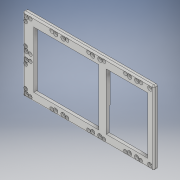
# Autodesk Inventor part: 30_CUBE_openSIM_Cagelid
Saved by Autodesk Inventor 2019 (Build 230136000, 136)
## iProperties
Created: 2020-08-12
Part Number: 30_CUBE_openSIM_Cagelid
Material: Generic
Document SubType Name: Modeling
Designer: wanghaoran
Density: 1 g/cm^3
Appearance: Default
Author: wanghaoran
Autodesk Inventor part; units mm, degrees
ref_plane "YZ Plane" through (0, 0, 0) normal (1, 0, 0) x (0, 1, 0)
ref_plane "XZ Plane" through (0, 0, 0) normal (0, 1, 0) x (-1, 0, 0)
ref_plane "XY Plane" through (0, 0, 0) normal (0, 0, 1) x (1, 0, 0)
sketch "Sketch1" plane through (0, 0, 0) normal (0, 0, 1) x (1, 0, 0)
  line L0 (0, 0) -> (177.7, 0)
  line L1 (177.7, 0) -> (177.7, 99.8)
  line L2 (177.7, 99.8) -> (0, 99.8)
  line L3 (0, 99.8) -> (0, 0)
  dimension "d0" = 177.7
  dimension "d1" = 99.8
  constraints: 8 end point, 2 parallel, 1 horizontal, 1 perpendicular
  measures "d0" distance of L2.end L1.end
  measures "d1" distance of L1.end L0.end
extrude "Extrusion1" add sketch "Sketch1" along normal blind 5.079
sketch "Sketch3" plane through (0, 0, 5.079) normal (0, 0, 1) x (1, 0, 0)
  circle A0 centre (172.7, 94.9) radius 1.45 projected
  circle A1 centre (104.9, 94.9) radius 1.45 projected
  circle A2 centre (4.9, 94.9) radius 1.45 projected
  circle A3 centre (4.9, 4.9) radius 1.6 projected
  circle A4 centre (172.7, 4.9) radius 1.45 projected
  circle A5 centre (4.9, 44.9) radius 1.6 projected
  arc A6 (144.1319, 97.8) -> (145.6681, 97.8) centre (144.9, 94.9) ccw projected
  arc A7 (154.1319, 97.8) -> (155.6681, 97.8) centre (154.9, 94.9) ccw projected
  arc A8 (94.1319, 97.8) -> (95.6681, 97.8) centre (94.9, 94.9) ccw projected
  arc A9 (54.1319, 97.8) -> (55.6681, 97.8) centre (54.9, 94.9) ccw projected
  arc A10 (44.1319, 97.8) -> (45.6681, 97.8) centre (44.9, 94.9) ccw projected
  arc A11 (2, 54.1319) -> (2, 55.6681) centre (4.9, 54.9) ccw projected
  arc A12 (2, 44.1319) -> (2, 45.6681) centre (4.9, 44.9) ccw projected
  arc A13 (45.6681, 2) -> (44.1319, 2) centre (44.9, 4.9) ccw projected
  arc A14 (55.6681, 2) -> (54.1319, 2) centre (54.9, 4.9) ccw projected
  arc A15 (95.6681, 2) -> (94.1319, 2) centre (94.9, 4.9) ccw projected
  arc A16 (105.6681, 2) -> (104.1319, 2) centre (104.9, 4.9) ccw projected
  arc A17 (145.6681, 2) -> (144.1319, 2) centre (144.9, 4.9) ccw projected
  arc A18 (155.6681, 2) -> (154.1319, 2) centre (154.9, 4.9) ccw projected
hole "Hole1" at (172.7, 4.9, 5.079) at (172.7, 94.9, 5.079) at (4.9, 94.9, 5.079) at (4.9, 44.9, 5.079) at (4.9, 4.9, 5.079) at (144.9, 94.9, 5.079) at (154.9, 94.9, 5.079) at (154.9, 4.9, 5.079) at (144.9, 4.9, 5.079) at (104.9, 4.9, 5.079) at (94.9, 4.9, 5.079) at (104.9, 94.9, 5.079) at (94.9, 94.9, 5.079) at (54.9, 94.9, 5.079) at (44.9, 94.9, 5.079) at (54.9, 4.9, 5.079) at (44.9, 4.9, 5.079) at (4.9, 54.9, 5.079) direction (0, 0, -1) diameter 2.9 depth 12 tip angle 118 counterbore diameter 6 counterbore depth 2.5
sketch "Sketch5" plane through (0, 0, 0) normal (0, 0, -1) x (-1, 0, 0)
  line L0 (-15, 11.5) -> (-169.7, 11.5)
  line L1 (-169.7, 11.5) -> (-169.7, 88.3)
  line L2 (-169.7, 88.3) -> (-15, 88.3)
  line L3 (-15, 88.3) -> (-15, 11.5)
  line L4 (0, 99.8) -> (0, 0) projected
  line L5 (-103.5, 88.3) -> (-113.5, 88.3)
  line L6 (-113.5, 88.3) -> (-113.5, 11.5)
  line L7 (-113.5, 11.5) -> (-103.5, 11.5)
  line L8 (-103.5, 11.5) -> (-103.5, 88.3)
  dimension "d28" = 154.7
  dimension "d29" = 76.8
  dimension "d49" = 15
  dimension "d58" = 10
  dimension "d59" = 76.8
  dimension "d60" = 56.2
  constraints: 16 end point, 4 parallel, 2 horizontal, 2 perpendicular, 1 point on line
  measures "d28" distance of L1.end L2.end
  measures "d29" distance of L0.end L1.end
  measures "d49" distance between parallel lines of L3 L4
  measures "d58" distance of L7.end L6.end
  measures "d59" distance of L6.end L5.end
  measures "d60" distance between parallel lines of L1 L6
extrude "Extrusion4" cut sketch "Sketch5" against normal through all contours L0 L8 L2 L3 | L0 L1 L2 L6
fillet "Fillet1" radius 2 8 edges at (88.85, 0, 5.079) (0, 49.9, 5.079) (177.7, 49.9, 5.079) (88.85, 99.8, 5.079) (177.7, 0, 2.5395) (177.7, 99.8, 2.5395) (0, 0, 2.5395) (0, 99.8, 2.5395)
sketch "Sketch7" plane through (103.5, 11.5, 0) normal (-1, 0, 0) x (0, 0, 1)
  circle A0 centre (-19.9999, 12.5) radius 13.3985 projected
  line L0 (-1.6569, 33.566) -> (-38.3429, 33.566)
  line L1 (-38.3429, 33.566) -> (-41.0659, 30.843)
  line L2 (-41.0659, 30.843) -> (-41.0659, -5.843)
  line L3 (-41.0659, -5.843) -> (-38.3429, -8.566)
  line L4 (-38.3429, -8.566) -> (-1.6569, -8.566)
  line L5 (-1.6569, -8.566) -> (1.0661, -5.843)
  line L6 (1.0661, -5.843) -> (1.0661, 30.843)
  line L7 (1.0661, 30.843) -> (-1.6569, 33.566)
  point P0 (0, -11.5)
  constraints: 16 end point
extrude "Extrusion6" cut sketch "Sketch7" against normal up to surface (154.7 mm away) from surface at 88.5
sketch "Sketch8" plane through (0, 0, 5.079) normal (0, 0, 1) x (1, 0, 0)
  circle A0 centre (160.4, 4.1) radius 2.65 projected
  circle A1 centre (189.4, 4.1) radius 2.65 projected
  circle A2 centre (154.1, 10.4) radius 2.65 projected
  circle A3 centre (195.7, 10.4) radius 2.65 projected
  circle A4 centre (145.7, 10.4) radius 2.65 projected
  circle A5 centre (139.4, 4.1) radius 2.65 projected
  circle A6 centre (110.4, 4.1) radius 2.65 projected
  circle A7 centre (89.4, 4.1) radius 2.65 projected
  circle A8 centre (60.4, 4.1) radius 2.65 projected
  circle A9 centre (39.4, 4.1) radius 2.65 projected
  circle A10 centre (10.4, 4.1) radius 2.65 projected
  circle A11 centre (4.1, 10.4) radius 2.65 projected
  circle A12 centre (4.1, 39.4) radius 2.65 projected
  circle A13 centre (10.4, 45.7) radius 2.65 projected
  circle A14 centre (4.1, 89.4) radius 2.65 projected
  circle A15 centre (10.4, 95.7) radius 2.65 projected
  circle A16 centre (39.4, 95.7) radius 2.65 projected
  circle A17 centre (60.4, 95.7) radius 2.65 projected
  circle A18 centre (89.4, 95.7) radius 2.65 projected
  circle A19 centre (110.4, 95.7) radius 2.65 projected
  circle A20 centre (139.4, 95.7) radius 2.65 projected
  circle A21 centre (160.4, 95.7) radius 2.65 projected
  circle A22 centre (189.4, 95.7) radius 2.65 projected
  circle A23 centre (4.1, 60.4) radius 2.65 projected
  circle A24 centre (10.4, 54.1) radius 2.65 projected
  circle A25 centre (4.1, 89.4) radius 2.45
  circle A26 centre (10.4, 95.7) radius 2.45
  circle A27 centre (4.1, 60.4) radius 2.45
  circle A28 centre (10.4, 54.1) radius 2.45
  circle A29 centre (10.4, 45.7) radius 2.45
  circle A30 centre (4.1, 39.4) radius 2.45
  circle A31 centre (4.1, 10.4) radius 2.45
  circle A32 centre (10.4, 4.1) radius 2.45
  circle A33 centre (39.4, 4.1) radius 2.45
  line L0 (103.5, 11.5) -> (15, 11.5) projected
  line L1 (15, 11.5) -> (25, 11.5)
  circle A34 centre (60.4, 4.1) radius 2.45
  circle A35 centre (89.4, 4.1) radius 2.45
  circle A36 centre (110.4, 4.1) radius 2.45
  circle A37 centre (139.4, 4.1) radius 2.45
  circle A38 centre (160.4, 4.1) radius 2.45
  circle A39 centre (160.4, 95.7) radius 2.45
  circle A40 centre (139.4, 95.7) radius 2.45
  circle A41 centre (110.4, 95.7) radius 2.45
  circle A42 centre (89.4, 95.7) radius 2.45
  circle A43 centre (60.4, 95.7) radius 2.45
  circle A44 centre (39.4, 95.7) radius 2.45
  point P0 (0, 0)
  dimension "d69" = 0.2
  dimension "d70" = 0.2
  dimension "d71" = 4.9
  dimension "d72" = 4.9
  dimension "d73" = 4.9
  dimension "d74" = 4.9
  dimension "d75" = 4.9
  dimension "d76" = 4.9
  dimension "d77" = 4.9
  dimension "d85" = 4.9
  dimension "d86" = 4.9
  dimension "d87" = 4.9
  dimension "d88" = 4.9
  dimension "d89" = 4.9
  dimension "d90" = 4.9
  dimension "d91" = 4.9
  dimension "d92" = 4.9
  dimension "d93" = 4.9
  dimension "d94" = 4.9
  dimension "d95" = 4.9
  constraints: 20 centre point, 18 coincident, 2 end point, 1 point on line
  measures "d69" radial gap between concentric circles of A14 A25
  measures "d70" radial gap between concentric circles of A15 A26
  measures "d71" diameter of A27
  measures "d72" diameter of A28
  measures "d73" diameter of A29
  measures "d74" diameter of A30
  measures "d75" diameter of A31
  measures "d76" diameter of A32
  measures "d77" diameter of A33
  measures "d85" diameter of A34
  measures "d86" diameter of A35
  measures "d87" diameter of A36
  measures "d88" diameter of A37
  measures "d89" diameter of A38
  measures "d90" diameter of A39
  measures "d91" diameter of A40
  measures "d92" diameter of A41
  measures "d93" diameter of A42
  measures "d94" diameter of A43
  measures "d95" diameter of A44
extrude "Extrusion8" cut sketch "Sketch8" against normal blind 10 contours A25 | A26 | A27 | A28 | A29 | A30 | A31 | A32 | A33 | A34 | A35 | A36 | A37 | A38 | A39 | A40 | A41 | A42 | A43 | A44
body "Solid1"
